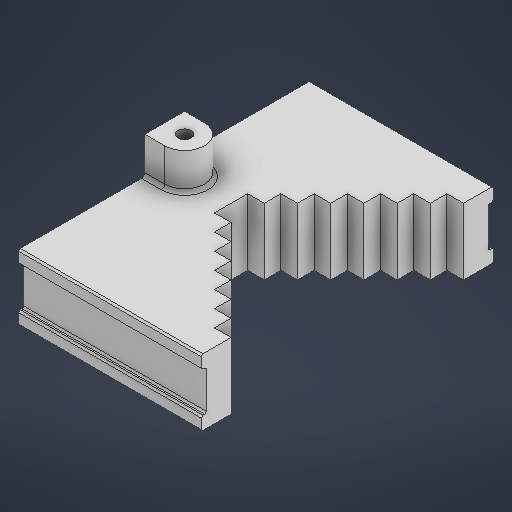
# Autodesk Inventor part: pfa
Saved by Autodesk Inventor 2026.1 (Build 301233000, 233)
## iProperties
Created: 2025-09-15
Part Number: pfa
Material: Generic
Document SubType Name: Modeling
Designer: student
Density: 1 g/cm^3
Appearance: Default
Author: student
Autodesk Inventor part; units mm, degrees
ref_plane "YZ Plane" through (0, 0, 0) normal (1, 0, 0) x (0, 1, 0)
ref_plane "XZ Plane" through (0, 0, 0) normal (0, 1, 0) x (-1, 0, 0)
ref_plane "XY Plane" through (0, 0, 0) normal (0, 0, 1) x (1, 0, 0)
sketch "Sketch1" plane through (0, 0, 0) normal (0, 1, 0) x (-1, 0, 0)
  line L0 (-27.5, 44) -> (27.5, 44)
  line L1 (27.5, 44) -> (27.5, -44)
  line L2 (27.5, -44) -> (-27.5, -44)
  line L3 (-27.5, -44) -> (-27.5, 44)
  line L4 (-27.5, 44) -> (27.5, -44) construction
  line L5 (27.5, 44) -> (-27.5, -44) construction
  line L6 (-27.5, 44) -> (-22.5, 44)
  line L7 (-22.5, 44) -> (-22.5, 35)
  line L8 (-22.5, 35) -> (-27.5, 35)
  line L9 (-27.5, 35) -> (-27.5, 44)
  line L10 (-22.5, 35) -> (-17.5, 35)
  line L11 (-17.5, 35) -> (-17.5, 30)
  line L12 (-17.5, 30) -> (-22.5, 30)
  line L13 (-22.5, 30) -> (-22.5, 35)
  line L14 (-17.5, 30) -> (-12.5, 30)
  line L15 (-12.5, 30) -> (-12.5, 25)
  line L16 (-12.5, 25) -> (-17.5, 25)
  line L17 (-17.5, 25) -> (-17.5, 30)
  line L18 (-12.5, 25) -> (-7.5, 25)
  line L19 (-7.5, 25) -> (-7.5, 20)
  line L20 (-7.5, 20) -> (-12.5, 20)
  line L21 (-12.5, 20) -> (-12.5, 25)
  line L22 (-7.5, 20) -> (-2.5, 20)
  line L23 (-2.5, 20) -> (-2.5, 15)
  line L24 (-2.5, 15) -> (-7.5, 15)
  line L25 (-7.5, 15) -> (-7.5, 20)
  line L26 (-2.5, 15) -> (2.5, 15)
  line L27 (2.5, 15) -> (2.5, 10)
  line L28 (2.5, 10) -> (-2.5, 10)
  line L29 (-2.5, 10) -> (-2.5, 15)
  line L30 (2.5, 10) -> (7.5, 10)
  line L31 (7.5, 10) -> (7.5, 5)
  line L32 (7.5, 5) -> (2.5, 5)
  line L33 (2.5, 5) -> (2.5, 10)
  line L34 (13, 5) -> (13, 0)
  line L35 (13, 0) -> (8, 0)
  line L36 (8, 0) -> (8, 5)
  line L37 (-27.5, -44) -> (27.5, 44) construction
  line L38 (-22.5, -35) -> (-27.5, -35)
  line L39 (-17.5, -30) -> (-22.5, -30)
  line L40 (-22.5, -30) -> (-22.5, -35)
  line L41 (-17.5, -25) -> (-17.5, -30)
  line L42 (-7.5, -20) -> (-12.5, -20)
  line L43 (-12.5, -20) -> (-12.5, -25)
  line L44 (-2.5, -15) -> (-7.5, -15)
  line L45 (-7.5, -15) -> (-7.5, -20)
  line L46 (2.5, -10) -> (-2.5, -10)
  line L47 (-2.5, -10) -> (-2.5, -15)
  line L48 (7.5, -5) -> (2.5, -5)
  line L49 (2.5, -5) -> (2.5, -10)
  line L50 (8, 0) -> (8, -5)
  line L51 (7.5, 5) -> (7.5, -5)
  line L52 (27.5, 0) -> (21.5, 0)
  circle A0 centre (21.5, 0) radius 6
  line L53 (-12.5, -25) -> (-17.5, -25)
  point P0 (0, 0)
  dimension "d0" = 55
  dimension "d1" = 88
  dimension "d2" = 5
  dimension "d3" = 9
  dimension "d4" = 5
  dimension "d5" = 5
  dimension "d6" = 5
  dimension "d7" = 5
  dimension "d8" = 5
  dimension "d9" = 5
  dimension "d10" = 5
  dimension "d11" = 5
  dimension "d12" = 5
  dimension "d13" = 5
  dimension "d14" = 5
  dimension "d15" = 5
  dimension "d16" = 5
  dimension "d17" = 5
  dimension "d18" = 6
  constraints: 108 end point, 17 parallel, 16 symmetric about line, 10 horizontal, 8 perpendicular, 3 midpoint, 3 point on line, 1 coincident, 1 horizontal alignment, 1 vertical, 2 other
  measures "d0" distance of L1.end L2.end
  measures "d1" distance of L0.end L1.end
  measures "d2" distance of L7.end L8.end
  measures "d3" distance of L6.end L7.end
  measures "d4" distance of L11.end L12.end
  measures "d5" distance of L10.end L11.end
  measures "d6" distance of L15.end L16.end
  measures "d7" distance of L14.end L15.end
  measures "d8" distance of L19.end L20.end
  measures "d9" distance of L18.end L19.end
  measures "d10" distance of L23.end L24.end
  measures "d11" distance of L22.end L23.end
  measures "d12" distance of L27.end L28.end
  measures "d13" distance of L26.end L27.end
  measures "d14" distance of L31.end L32.end
  measures "d15" distance of L30.end L31.end
  measures "d16" distance of L34.end L35.end
  measures "d17" distance of L34.start L34.end
  measures "d18" distance of L52.start L52.end
extrude "Extrusion1" add sketch "Sketch1" along normal blind 20 contours L0 L7 L8 L3 | A0 | L0 L1 L2 L3 L38 L40 L39 L41 L53 L43 L42 L45 L44 L47 L46 L49 L48 L51 L31 L30 L27 L26 L23 L22 L19 L18 L15 L14 L11 L10 L7 | L10 L11 L12 L13 | L14 L15 L16 L17 | L18 L19 L20 L21 | L22 L23 L24 L25 | L26 L27 L28 L29 | L30 L31 L32 L33
sketch "Sketch2" plane through (0, 0, 0) normal (0, -1, 0) x (1, 0, 0)
  line L0 (-27.5, -44) -> (-27.5, 44) projected
  line L1 (-27.5, 0) -> (-21.5, 0)
  circle A0 centre (-21.5, 0) radius 6
  line L2 (-21.5, -6) -> (-27.5, -6)
  line L3 (-21.5, 6) -> (-27.5, 6)
  point P0 (0, 0)
  dimension "d21" = 6
  constraints: 6 end point, 3 point on circle, 2 perpendicular, 2 point on line, 2 tangent, 1 centre point, 1 coincident, 1 horizontal, 1 midpoint
  measures "d21" distance of L1.start L1.end
extrude "Extrusion2" add sketch "Sketch2" along normal blind 11
sketch "Sketch3" plane through (0, 20, 0) normal (0, 1, 0) x (1, 0, 0)
  line L0 (-21.5, -6) -> (-27.5, -6) projected
  line L1 (-27.5, -6) -> (-27.5, 6) projected
  line L2 (-27.5, 6) -> (-21.5, 6) projected
  arc A0 (-21.5, -6) -> (-21.5, 6) centre (-21.5, 0) ccw projected
  point P0 (0, 0)
extrude "Extrusion3" add sketch "Sketch3" along normal blind 11
sketch "Sketch4" plane through (0, 31, 0) normal (0, 1, 0) x (1, 0, 0)
  arc A0 (-21.5, -6) -> (-21.5, 6) centre (-21.5, 0) ccw projected
  circle A1 centre (-21.5, 0) radius 2
  point P0 (0, 0)
  dimension "d26" = 4
  constraints: 1 centre point, 1 coincident
  measures "d26" diameter of A1
extrude "Extrusion4" cut sketch "Sketch4" against normal through all
sketch "Sketch5" plane through (-27.5, 0, 44) normal (-1, 0, 0) x (0, 0, 1)
  line L0 (-44, 0) -> (-44, 10)
  line L1 (-46, 31) -> (-46, -11) projected
  constraints: 2 end point, 1 parallel
hole "Hole1" at (-27.5, 10, 0) direction (1, 0, 0) diameter 16 depth 10 tip angle 118
sketch "Sketch6" plane through (-27.5, 0, 44) normal (-1, 0, 0) x (0, 0, 1)
  line L0 (1.5, 16) -> (-1.5, 16)
  line L1 (-1.5, 16) -> (-1.5, 4)
  line L2 (-1.5, 4) -> (1.5, 4)
  line L3 (1.5, 4) -> (1.5, 16)
  line L4 (0, 0) -> (0, 20) projected
  line L5 (1.5, 16) -> (-1.5, 4) construction
  line L6 (-1.5, 16) -> (1.5, 4) construction
  line L7 (-89.5, 16) -> (-86.5, 16)
  line L8 (-86.5, 16) -> (-86.5, 4)
  line L9 (-86.5, 4) -> (-89.5, 4)
  line L10 (-89.5, 4) -> (-89.5, 16)
  line L11 (-88, 0) -> (-88, 20) projected
  line L12 (-89.5, 16) -> (-86.5, 4) construction
  line L13 (-86.5, 16) -> (-89.5, 4) construction
  point P0 (-44, 0)
  point P1 (0, 10)
  point P2 (-88, 10)
  dimension "d36" = 3
  dimension "d37" = 12
  dimension "d38" = 3
  dimension "d39" = 12
  constraints: 24 end point, 6 midpoint, 4 parallel, 2 horizontal, 2 perpendicular
  measures "d36" distance of L2.end L1.end
  measures "d37" distance of L1.end L0.end
  measures "d38" distance of L8.end L9.end
  measures "d39" distance of L7.end L8.end
extrude "Extrusion5" cut sketch "Sketch6" against normal through all
fillet "Fillet1" radius 0.5 4 edges at (0, 4, 42.5) (0, 16, 42.5) (0, 4, -42.5) (0, 16, -42.5)
fillet "Fillet2" radius 1 6 edges at (-24.5, 20, -6) (-15.5, 20, 0) (-24.5, 20, 6) (-15.5, 0, 0) (-24.5, 0, 6) (-24.5, 0, -6)
chamfer "Chamfer1" distance 0.5 angle 45 8 edges at (0, 20, -44) (0, 16, -44) (0, 4, -44) (0, 0, -44) (0, 20, 44) (0, 16, 44) (0, 0, 44) (0, 4, 44)
thread "Thread1" size "M4x0.7" class "6H" standard "ANSI Metric M Profile" full length
thread "Thread2" size "M4x0.7" class "6H" standard "ANSI Metric M Profile" full length
body "Solid1"
